Autodesk Inventor part; units mm, degrees
(part 3 of 3)
  line L647 (29.016, 41.0123) -> (30.8387, 39.6618)
  line L648 (30.8387, 39.6618) -> (30.6085, 39.351)
  line L649 (30.6085, 39.351) -> (27.8288, 38.4441)
  line L650 (27.8288, 38.4441) -> (29.2148, 37.4173)
  line L651 (29.2148, 37.4173) -> (28.943, 37.0505)
  spline S498 degree 2 poles (32.4837, 36.267) (31.9739, 35.6622) (30.7657, 35.4182) (30.3234, 35.791) knots 0 0 0 1 2 2 2
  spline S499 degree 2 poles (30.3234, 35.791) (30.1236, 35.9595) (29.9216, 36.2983) (29.8549, 36.5004) knots 0 0 0 1 2 2 2
  line L652 (29.8549, 36.5004) -> (29.7317, 36.4083)
  line L653 (29.7317, 36.4083) -> (29.3427, 36.7362)
  line L654 (29.3427, 36.7362) -> (32.2375, 40.1705)
  line L655 (32.2375, 40.1705) -> (32.6532, 39.8202)
  line L656 (32.6532, 39.8202) -> (31.6201, 38.5946)
  spline S500 degree 2 poles (31.6201, 38.5946) (31.8963, 38.6033) (32.4185, 38.4821) (32.6503, 38.2867) knots 0 0 0 1 2 2 2
  spline S501 degree 2 poles (32.6503, 38.2867) (33.0686, 37.9341) (32.9845, 36.8611) (32.4837, 36.267) knots 0 0 0 1 2 2 2
  spline S502 degree 2 poles (32.0278, 36.5966) (32.4006, 37.0389) (32.5178, 37.724) (32.2194, 37.9755) knots 0 0 0 1 2 2 2
  spline S503 degree 2 poles (32.2194, 37.9755) (32.0515, 38.117) (31.5704, 38.2491) (31.3259, 38.2455) knots 0 0 0 1 2 2 2
  line L657 (31.3259, 38.2455) -> (30.1334, 36.8308)
  spline S504 degree 2 poles (30.1334, 36.8308) (30.2254, 36.621) (30.414, 36.3527) (30.5579, 36.2314) knots 0 0 0 1 2 2 2
  spline S505 degree 2 poles (30.5579, 36.2314) (30.8749, 35.9642) (31.6168, 36.109) (32.0278, 36.5966) knots 0 0 0 1 2 2 2
  line L658 (33.6246, 32.8627) -> (33.2344, 33.2412)
  line L659 (33.2344, 33.2412) -> (33.4819, 33.4963)
  spline S506 degree 2 poles (33.4819, 33.4963) (33.149, 33.5134) (32.6686, 33.6638) (32.4685, 33.8579) knots 0 0 0 1 2 2 2
  spline S507 degree 2 poles (32.4685, 33.8579) (32.3184, 34.0035) (32.1479, 34.3632) (32.1546, 34.5653) knots 0 0 0 1 2 2 2
  spline S508 degree 2 poles (32.1546, 34.5653) (32.1589, 34.7699) (32.3667, 35.2043) (32.5947, 35.4395) knots 0 0 0 1 2 2 2
  line L660 (32.5947, 35.4395) -> (34.0529, 36.9427)
  line L661 (34.0529, 36.9427) -> (34.4431, 36.5642)
  line L662 (34.4431, 36.5642) -> (33.162, 35.2436)
  spline S509 degree 2 poles (33.162, 35.2436) (32.9825, 35.0585) (32.7747, 34.7892) (32.7349, 34.653) knots 0 0 0 1 2 2 2
  spline S510 degree 2 poles (32.7349, 34.653) (32.695, 34.5169) (32.7776, 34.2766) (32.9301, 34.1286) knots 0 0 0 1 2 2 2
  spline S511 degree 2 poles (32.9301, 34.1286) (33.0727, 33.9904) (33.5531, 33.84) (33.8022, 33.8265) knots 0 0 0 1 2 2 2
  line L663 (33.8022, 33.8265) -> (35.4811, 35.5573)
  line L664 (35.4811, 35.5573) -> (35.8713, 35.1789)
  line L665 (35.8713, 35.1789) -> (33.6246, 32.8627)
  line L666 (37.2668, 32.8158) -> (37.2479, 32.8363)
  spline S512 degree 2 poles (37.2479, 32.8363) (37.2183, 32.8943) (37.1315, 32.9991) (37.0679, 33.0684) knots 0 0 0 1 2 2 2
  spline S513 degree 2 poles (37.0679, 33.0684) (36.9194, 33.2301) (36.4859, 33.4187) (36.2154, 33.4351) knots 0 0 0 1 2 2 2
  line L667 (36.2154, 33.4351) -> (34.5292, 31.8865)
  line L668 (34.5292, 31.8865) -> (34.1615, 32.2869)
  line L669 (34.1615, 32.2869) -> (36.538, 34.4695)
  line L670 (36.538, 34.4695) -> (36.9057, 34.0692)
  line L671 (36.9057, 34.0692) -> (36.5516, 33.7439)
  spline S514 degree 2 poles (36.5516, 33.7439) (36.947, 33.7049) (37.4054, 33.5251) (37.5469, 33.3711) knots 0 0 0 1 2 2 2
  spline S515 degree 2 poles (37.5469, 33.3711) (37.6034, 33.3095) (37.6549, 33.2432) (37.6825, 33.1976) knots 0 0 0 1 2 2 2
  line L672 (37.6825, 33.1976) -> (37.2668, 32.8158)
  spline S516 degree 2 poles (35.2727, 30.2967) (35.2891, 30.2381) (35.3643, 30.025) (35.4261, 29.9) knots 0 0 0 1 2 2 2
  spline S517 degree 2 poles (35.4261, 29.9) (35.4913, 29.7597) (35.6172, 29.5341) (35.7121, 29.4181) knots 0 0 0 1 2 2 2
  spline S518 degree 2 poles (35.7121, 29.4181) (35.8709, 29.2239) (36.194, 29.0379) (36.3475, 29.0374) knots 0 0 0 1 2 2 2
  spline S519 degree 2 poles (36.3475, 29.0374) (36.4987, 29.0396) (36.7851, 29.1792) (36.9389, 29.305) knots 0 0 0 1 2 2 2
  line L673 (36.9389, 29.305) -> (37.1574, 29.4836)
  spline S520 degree 2 poles (37.1574, 29.4836) (36.8701, 29.5323) (36.4629, 29.744) (36.2622, 29.9895) knots 0 0 0 1 2 2 2
  spline S521 degree 2 poles (36.2622, 29.9895) (35.9136, 30.4157) (36.1351, 31.4385) (36.7312, 31.926) knots 0 0 0 1 2 2 2
  spline S522 degree 2 poles (36.7312, 31.926) (37.0415, 32.1796) (37.665, 32.3969) (37.9541, 32.3902) knots 0 0 0 1 2 2 2
  spline S523 degree 2 poles (37.9541, 32.3902) (38.2279, 32.3801) (38.7187, 32.1377) (38.8863, 31.9327) knots 0 0 0 1 2 2 2
  spline S524 degree 2 poles (38.8863, 31.9327) (39.0452, 31.7385) (39.1851, 31.3802) (39.2183, 31.1689) knots 0 0 0 1 2 2 2
  line L674 (39.2183, 31.1689) -> (39.3434, 31.2306)
  line L675 (39.3434, 31.2306) -> (39.6677, 30.8341)
  line L676 (39.6677, 30.8341) -> (37.4557, 29.0253)
  spline S525 degree 2 poles (37.4557, 29.0253) (36.819, 28.5048) (35.7734, 28.5725) (35.3079, 29.1417) knots 0 0 0 1 2 2 2
  spline S526 degree 2 poles (35.3079, 29.1417) (35.158, 29.3251) (34.9041, 29.7567) (34.8181, 29.9609) knots 0 0 0 1 2 2 2
  line L677 (34.8181, 29.9609) -> (35.2551, 30.3183)
  line L678 (35.2551, 30.3183) -> (35.2727, 30.2967)
  line L679 (37.5027, 29.766) -> (38.8758, 30.8888)
  spline S527 degree 2 poles (38.8758, 30.8888) (38.8233, 31.107) (38.6719, 31.4243) (38.5638, 31.5565) knots 0 0 0 1 2 2 2
  spline S528 degree 2 poles (38.5638, 31.5565) (38.3035, 31.8748) (37.5342, 31.8578) (37.0945, 31.4983) knots 0 0 0 1 2 2 2
  spline S529 degree 2 poles (37.0945, 31.4983) (36.6791, 31.1586) (36.4719, 30.5256) (36.7278, 30.2127) knots 0 0 0 1 2 2 2
  spline S530 degree 2 poles (36.7278, 30.2127) (36.8624, 30.0481) (37.2742, 29.8087) (37.5027, 29.766) knots 0 0 0 1 2 2 2
  point P0 (0, 0)
  constraints: 1 other
extrude "Extrusion2" add sketch "Skizze2" along normal blind 1 contours L0 L1 L2 L3 L4 L5 L6 L7 L8 L9 L10 L11 | L12 L13 L14 L15 L16 L17 L18 L19 L20 L21 L22 L23 | L24 L25 L26 L27 L28 L29 L30 L31 L32 L33 L34 L35 | L36 L37 L38 L39 L40 L41 L42 L43 L44 L45 L46 L47 L48 L49 L50 L51 L52 L53 L54 L55 L56 L57 L58 L59 L60 L61 L62 L63 | S0 S1 L68 L69 L70 L71 L72 S2 S3 | L74 L75 L76 L77 | L78 L79 L80 L81 | L82 S8 S9 S10 S11 L83 L84 L85 S12 S13 S14 L86 L87 L88 L89 L90 S15 S16 S17 S18 S19 L91 L92 | S20 S21 L93 L94 L95 L96 L97 S22 S23 | L99 L100 L101 L102 L103 L104 L105 L106 | S28 S29 S30 S31 | L107 L108 S36 S37 S38 L109 L110 L111 S39 S40 S41 L112 L113 L114 | L115 S42 S43 L116 L117 L118 L119 L120 S44 S45 L121 | S46 S47 L122 L123 L124 L125 L126 S48 S49 | L128 S54 S55 L129 L130 L131 L132 L133 S56 S57 L134 | L135 L136 L137 L138 | L139 L140 L141 L142 | L143 L144 S58 S59 S60 L145 L146 L147 L148 L149 S61 S62 L150 | S63 L151 L152 L153 L154 L155 L156 L157 L158 L159 L160 L161 S64 S65 S66 L162 L163 S67 | L164 L165 L166 L167 L168 L169 L170 L171 L172 L173 L174 L175 | L176 L177 L178 L179 L180 L181 L182 L183 L184 L185 L186 L187 | L188 L189 L190 L191 L192 L193 L194 L195 L196 L197 L198 L199 | L200 L201 L202 L203 L204 L205 L206 L207 L208 L209 L210 L211 L212 | S68 S69 S70 S71 L213 L214 S72 S73 S74 L215 L216 S75 S76 | L218 S81 S82 S83 S84 L219 L220 L221 S85 S86 S87 L222 L223 L224 L225 L226 S88 S89 S90 S91 S92 L227 L228 | S93 S94 L229 L230 L231 L232 L233 S95 S96 | L235 S101 S102 L236 L237 L238 L239 L240 S103 S104 L241 | S105 S106 S107 S108 S109 S110 L242 S111 S112 S113 L243 L244 S114 S115 S116 L245 L246 L247 | L249 L250 S121 S122 S123 L251 L252 L253 L254 L255 S124 S125 L256 | S126 S127 S128 S129 L257 L258 S130 S131 S132 L259 L260 S133 S134 | S139 S140 L262 L263 L264 S141 S142 S143 L265 S144 | L272 L273 L274 L275 | L276 L277 L278 L279 | S153 S154 S155 S156 | S161 S162 L280 L281 L282 L283 L284 S163 S164 | L286 L287 S169 S170 S171 L288 L289 L290 L291 L292 S172 S173 L293 | L294 L295 L296 L297 L298 L299 L300 L301 | S174 L302 L303 S175 S176 S177 S178 S179 S180 S181 S182 S183 L304 L305 S184 S185 S186 S187 S188 S189 S190 | L306 L307 L308 L309 | L310 L311 L312 L313 | S191 S192 S193 S194 S195 L314 L315 S196 S197 S198 S199 S200 L316 L317 S201 S202 | S203 L318 L319 S204 S205 S206 S207 S208 S209 S210 S211 S212 L320 L321 S213 S214 S215 S216 S217 S218 S219 | L322 L323 L324 L325 L326 L327 L328 L329 L330 L331 L332 L333 | L334 L335 L336 L337 L338 L339 L340 L341 L342 L343 L344 L345 | L346 L347 L348 L349 L350 L351 L352 L353 L354 L355 L356 L357 | L358 L359 L360 L361 L362 L363 L364 L365 L366 L367 L368 L369 L370 | S220 S221 S222 S223 | L371 S228 S229 L372 L373 L374 L375 L376 S230 S231 L377 | S232 S233 L378 L379 L380 L381 L382 S234 S235 | L384 L385 S240 S241 S242 L386 L387 L388 L389 L390 S243 S244 L391 | S245 S246 S247 S248 | S253 S254 L392 L393 L394 L395 L396 S255 S256 | L400 L401 S261 S262 S263 L402 L403 L404 L405 L406 S264 S265 L407 | L408 L409 L410 L411 L412 L413 L414 L415 | S266 L416 L417 S267 S268 S269 S270 S271 S272 S273 S274 S275 L418 L419 S276 S277 S278 S279 S280 S281 S282 | L420 L421 L422 L423 | L424 L425 L426 L427 | S283 S284 S285 S286 S287 L428 L429 S288 S289 S290 S291 S292 L430 L431 S293 S294 | S295 L432 L433 S296 S297 S298 S299 S300 S301 S302 S303 S304 L434 L435 S305 S306 S307 S308 S309 S310 S311 | L436 L437 L438 L439 L440 L441 L442 L443 L444 L445 L446 L447 | L448 L449 L450 L451 L452 L453 L454 L455 L456 L457 L458 L459 | L460 L461 L462 L463 L464 L465 L466 L467 L468 L469 L470 L471 | S312 S313 L472 L473 L474 L475 L476 S314 S315 | S320 S321 S322 S323 S324 S325 L480 S326 S327 S328 L481 L482 S329 S330 S331 L483 L484 L485 | L487 S336 S337 L488 L489 L490 L491 L492 S338 S339 L493 | L494 L495 L496 L497 | L498 L499 L500 L501 | S340 L502 L503 S341 S342 S343 S344 S345 S346 S347 S348 S349 L504 L505 S350 S351 S352 S353 S354 S355 S356 | L506 L507 L508 L509 L510 L511 | S357 S358 S359 S360 | L512 L513 S365 S366 S367 S368 S369 S370 S371 L514 L515 L516 | L518 S376 S377 L519 L520 L521 L522 L523 S378 S379 L524 | S380 S381 S382 S383 | L525 L526 S388 S389 S390 L527 L528 L529 L530 L531 S391 S392 L532 | S393 S394 L533 L534 L535 S395 S396 S397 S398 L536 L537 L538 S399 S400 | L539 L540 S401 S402 S403 L541 L542 L543 L544 L545 S404 S405 L546 | L547 L548 L549 L550 | L551 L552 L553 L554 | L555 L556 L557 L558 L559 L560 L561 | S406 S407 S408 S409 L562 L563 S410 S411 S412 L564 L565 S413 S414 | L567 S419 S420 L568 L569 L570 L571 L572 S421 S422 L573 | S423 L574 L575 S424 S425 S426 S427 S428 S429 S430 S431 S432 L576 L577 S433 S434 S435 S436 S437 S438 S439 | L578 L579 L580 L581 | L582 L583 L584 L585 | S440 L586 L587 L588 L589 L590 L591 L592 L593 L594 L595 L596 S441 S442 S443 L597 L598 S444 | S445 S446 S447 S448 S449 S450 L599 S451 S452 S453 L600 L601 S454 S455 S456 L602 L603 L604 | L606 L607 L608 L609 | L610 L611 L612 L613 | S461 L614 L615 L616 L617 L618 L619 L620 L621 L622 L623 L624 S462 S463 S464 L625 L626 S465 | S466 L627 L628 S467 S468 S469 S470 S471 S472 S473 S474 L629 L630 S475 S476 S477 S478 S479 S480 S481 | S482 S483 S484 S485 S486 S487 L631 S488 S489 S490 L632 L633 S491 S492 S493 L634 L635 L636 | L638 L639 L640 L641 | L642 L643 L644 L645 L646 L647 L648 L649 L650 L651 | S498 S499 L652 L653 L654 L655 L656 S500 S501 | L658 L659 S506 S507 S508 L660 L661 L662 S509 S510 S511 L663 L664 L665 | L666 S512 S513 L667 L668 L669 L670 L671 S514 S515 L672 | S516 S517 S518 S519 L673 S520 S521 S522 S523 S524 L674 L675 L676 S525 S526 L677 L678
fillet "Rundung2" radius 2 16 edges at (-55, 4, 0) (55, 4, 0) (5, 4, 57.3861) (-5, 4, 57.3861) (-12, 4, 62.5) (-7.25, 4, 60) (12, 4, 62.5) (7.25, 4, 60) (0, 4, 65) (-12, 4, -62.5) (-7.25, 4, -60) (12, 4, -62.5) (7.25, 4, -60) (0, 4, -65) (-5, 4, -57.3861) (5, 4, -57.3861)
ref_plane "Arbeitsebene1" through (0, 0, 0) normal (0, 0, 1) x (1, 0, 0)
